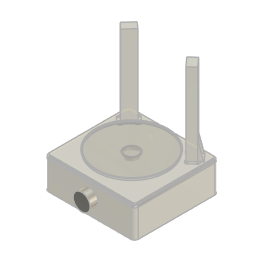
Elegoo Mercury X Cure Station (Autodesk Fusion 360 design; units mm, degrees)
Autodesk Fusion 360 part; units mm, degrees
sketch "Base" plane through (0, 0, 0) normal (0, 0, 1) x (1, 0, 0)
  line L0 (-113, 115) -> (113, 115)
  line L1 (123, 105) -> (123, -105)
  line L2 (113, -115) -> (-113, -115)
  line L3 (-123, -105) -> (-123, 105)
  arc A0 (-113, 115) -> (-123, 105) centre (-113, 105) ccw
  arc A1 (123, 105) -> (113, 115) centre (113, 105) ccw
  arc A2 (113, -115) -> (123, -105) centre (113, -105) ccw
  arc A3 (-123, -105) -> (-113, -115) centre (-113, -105) ccw
  line L4 (-113, 105) -> (113, -105) construction
  dimension "d1" = 10
  dimension "d7" = 246
  dimension "d8" = 230
  constraint horizontal L0
  constraint vertical L1
  constraint horizontal L2
  constraint vertical L3
  constraint tangent L0 A0
  constraint tangent L3 A0
  constraint tangent L0 A1
  constraint tangent L1 A1
  constraint equal A0 A1
  constraint tangent L1 A2
  constraint tangent L2 A2
  constraint equal A0 A2
  constraint tangent L2 A3
  constraint tangent L3 A3
  constraint equal A0 A3
  constraint coincident A0.centre L4.start
  constraint coincident A2.centre L4.end
  constraint midpoint origin L4
  measures "d1" radius of A0
  measures "d7" distance of L1 L3
  measures "d8" distance of L0 L2
extrude "Extrude1" add sketch "Base" along normal blind 81.5 makes body 1
sketch "Base Top" plane through (0, 0, 81.5) normal (0, 0, 1) x (-1, 0, 0)
  arc A0 (113, -115) -> (123, -105) centre (113, -105) ccw
  line L0 (123, -105) -> (123, 105)
  arc A1 (123, 105) -> (113, 115) centre (113, 105) ccw
  line L1 (113, 115) -> (-113, 115)
  arc A2 (-113, 115) -> (-123, 105) centre (-113, 105) ccw
  line L2 (-123, 105) -> (-123, -105)
  arc A3 (-123, -105) -> (-113, -115) centre (-113, -105) ccw
  line L3 (-113, -115) -> (113, -115)
  line L4 (113, 111) -> (-113, 111)
  arc A4 (-113, 111) -> (-119, 105) centre (-113, 105) ccw
  line L5 (-119, 105) -> (-119, -105)
  arc A5 (-119, -105) -> (-113, -111) centre (-113, -105) ccw
  line L6 (-113, -111) -> (113, -111)
  arc A6 (113, -111) -> (119, -105) centre (113, -105) ccw
  line L7 (119, -105) -> (119, 105)
  arc A7 (119, 105) -> (113, 111) centre (113, 105) ccw
  line L8 (113, 114.5) -> (-113, 114.5)
  arc A8 (-113, 114.5) -> (-122.5, 105) centre (-113, 105) ccw
  line L9 (-122.5, 105) -> (-122.5, -105)
  arc A9 (-122.5, -105) -> (-113, -114.5) centre (-113, -105) ccw
  line L10 (-113, -114.5) -> (113, -114.5)
  arc A10 (113, -114.5) -> (122.5, -105) centre (113, -105) ccw
  line L11 (122.5, -105) -> (122.5, 105)
  arc A11 (122.5, 105) -> (113, 114.5) centre (113, 105) ccw
  dimension "d53" = -0.5
  dimension "d54" = 3.5
  measures "d54" distance of L7 L11
extrude "Extrude2" add sketch "Base Top" along normal blind 4 contours L4 A4 L5 A5 L6 A6 L7 A7 bodies 1
extrude "Extrude8" cut sketch "Base Top" against normal blind 5.2 contours A0 L0 A1 L1 A2 L2 A3 L3 bodies 1
sketch "Wheel" plane through (0, -115, 0) normal (0, -1, 0) x (1, 0, 0)
  line L0 (-113, 0) -> (113, 0)
  line L1 (113, 0) -> (113, 76.3)
  line L2 (-113, 76.3) -> (-113, 0)
  circle A0 centre (0, 43.15) radius 23.35
  line L3 (0, 66.5) -> (0, 81.5) construction
  line L4 (113, 76.3) -> (-113, 76.3)
  dimension "d9" = 46.7
  dimension "d10" = 15
  constraint coincident A0 L3.start
  constraint vertical L3
  constraint coincident A0.centre L3
  measures "d9" diameter of A0
  measures "d10" distance of L3.start L3.end
extrude "Extrude3" add sketch "Wheel" along normal blind 22 contours A0 bodies 1
sketch "Plate" plane through (0, 0, 0) normal (0, 1, 0) x (1, 0, 0)
  line L0 (20.25, -81.275) -> (20.6, -94.275)
  line L1 (20.6, -94.275) -> (96.966, -94.275)
  line L2 (96.966, -94.275) -> (98.5, -100)
  line L3 (95.3809, -98.405) -> (0, -98.405)
  line L4 (0, -98.405) -> (0, -94.275)
  line L5 (0, -94.275) -> (17.4, -94.275)
  line L6 (17.4, -94.275) -> (17.75, -81.275)
  line L7 (17.75, -81.275) -> (20.25, -81.275)
  line L8 (98.5, -100) -> (95.8083, -100)
  line L9 (95.8083, -100) -> (95.3809, -98.405)
  line L10 (-113, -85.5) -> (113, -85.5)
  dimension "d14" = 98.5
  dimension "d16" = 2.6
  dimension "d17" = 5.725
  dimension "d18" = 4.13
  dimension "d20" = 20.6
  dimension "d23" = 20.25
  dimension "d24" = 2.5
  dimension "d25" = 13
  dimension "d27" = 75
  dimension "d28" = 14.5
  constraint perpendicular L3 L4
  constraint perpendicular L4 L5
  constraint horizontal L8
  constraint parallel L2 L9
  constraint horizontal L7
  constraint coincident L0.end L5
  constraint equal L0 L6
  constraint coincident origin L4
  measures "d14" distance of L4 L2.end
  measures "d16" distance of L2 L9
  measures "d17" distance of L1 L8
  measures "d18" distance of L1 L3
  measures "d20" distance of L0.end L4
  measures "d23" distance of L0.start L4
  measures "d24" distance of L0.start L6.end
  measures "d25" distance of L5.end L7
  measures "d27" angle of L1 L2
  measures "d28" distance of L8 L10
revolve "Revolve1" add sketch "Plate" angle 360 about axis through (0, 0, 98.405) along (0, 0, -1) separate body makes body 2
sketch "Tower" plane through (0, 0, 85.5) normal (0, 0, 1) x (-1, 0, 0)
  arc A0 (119, 105) -> (113, 111) centre (113, 105) ccw
  line L0 (113, 111) -> (-113, 111)
  arc A1 (-113, 111) -> (-119, 105) centre (-113, 105) ccw
  line L1 (-119, 105) -> (-119, -105)
  arc A2 (-119, -105) -> (-113, -111) centre (-113, -105) ccw
  line L2 (-113, -111) -> (113, -111)
  arc A3 (113, -111) -> (119, -105) centre (113, -105) ccw
  line L3 (119, -105) -> (119, 105)
  line L4 (89.4753, -59.2376) -> (106.3, -74.9248)
  line L5 (106.3, -74.9248) -> (84.3525, -99.3)
  line L6 (84.3525, -99.3) -> (66.9925, -84.2073)
  line L7 (66.9925, -84.2073) -> (89.4753, -59.2376)
  dimension "d30" = 32.8
  dimension "d31" = 33.6
  dimension "d32" = 23
  dimension "d33" = 12.7
  dimension "d34" = 11.7
  dimension "d36" = 42
  constraint parallel L5 L7
  constraint equal L4 L6
  measures "d30" distance of L4.end L5.end
  measures "d31" distance of L4.start L6.end
  measures "d32" distance of L5 L7
  measures "d33" distance of L3 L4.end
  measures "d34" distance of L2 L5.end
  measures "d36" angle of L3 L5
extrude "Extrude4" add sketch "Tower" along normal blind 225 separate body contours L4 L5 L6 L7 makes body 3
ref_plane "WorkPlane1" through (-86.6728, 79.3208, 198) normal (-0.669131, -0.743145, 0) x (0.743145, -0.669131, 0)
sketch "Tower Support" plane through (0.6366, 0.7071, 0) normal (-0.669131, -0.743145, 0) x (0.743145, -0.669131, 0)
  line L0 (-129.1308, 134.9) -> (-140.1308, 85.5)
  line L1 (-140.1308, 85.5) -> (-129.1308, 85.5)
  line L2 (-129.1308, 85.5) -> (-129.1308, 134.9)
  line L3 (-129.1308, 85.5) -> (-129.1308, 310.5)
  line L4 (-106.1308, 85.5) -> (-106.1308, 310.5)
  dimension "d39" = 34
  dimension "d40" = 49.4
  constraint horizontal L1
  constraint perpendicular L1 L2
  constraint coincident L0.start L3
  constraint coincident L1.end L2.start
  measures "d39" distance of L0.end L4
  measures "d40" distance of L0.start L1.end
extrude "Extrude5" add sketch "Tower Support" along normal mid plane 29 bodies 3
extrude "Extrude6" cut sketch "Tower Support" along normal mid plane 25.5 bodies 1 3
sketch "Tower Base" plane through (0, 0, 85.5) normal (0, 0, -1) x (1, 0, 0)
  line L0 (-112.0323, -84.9978) -> (-103.8577, -77.6373)
  line L1 (-103.8577, -77.6373) -> (-86.7948, -96.5875)
  line L2 (-86.7948, -96.5875) -> (-94.9694, -103.948)
  line L3 (-94.9694, -103.948) -> (-93.7985, -105.2485)
  line L4 (-93.7985, -105.2485) -> (-85.6239, -97.888)
  line L5 (-85.6239, -97.888) -> (-84.3525, -99.3)
  line L6 (-84.3525, -99.3) -> (-66.9925, -84.2073)
  line L7 (-66.9925, -84.2073) -> (-89.4753, -59.2376)
  line L8 (-89.4753, -59.2376) -> (-106.3, -74.9248)
  line L9 (-106.3, -74.9248) -> (-105.0287, -76.3368)
  line L10 (-105.0287, -76.3368) -> (-113.2032, -83.6973)
  line L11 (-113.2032, -83.6973) -> (-112.0323, -84.9978)
  line L12 (-93.84, -85.7742) -> (-88.3196, -91.9051)
  line L13 (-84.0828, -92.1272) -> (-71.0778, -80.4174)
  line L14 (-66.841, -80.6394) -> (-62.3578, -85.6185)
  line L15 (-62.5798, -89.8553) -> (-80.4153, -105.9144)
  line L16 (-84.6521, -105.6924) -> (-85.6224, -104.6148)
  line L17 (-89.8592, -104.3928) -> (-91.3455, -105.7311)
  line L18 (-95.5823, -105.509) -> (-104.6156, -95.4766)
  line L19 (-104.6156, -95.4766) -> (-93.84, -85.7742)
  circle A0 centre (-66.3041, -87.9607) radius 1.7
  circle A1 centre (-81.9102, -102.0125) radius 1.7
  circle A2 centre (-101.2714, -92.4655) radius 1.7
  line L20 (-81.9102, -102.0125) -> (-66.3041, -87.9607) construction
  arc A3 (-95.5823, -105.509) -> (-91.3455, -105.7311) centre (-93.3529, -103.5016) ccw
  arc A4 (-85.6224, -104.6148) -> (-89.8592, -104.3928) centre (-87.8518, -106.6222) ccw
  arc A5 (-84.6521, -105.6924) -> (-80.4153, -105.9144) centre (-82.4227, -103.685) ccw
  arc A6 (-62.5798, -89.8553) -> (-62.3578, -85.6185) centre (-64.5872, -87.6259) ccw
  arc A7 (-66.841, -80.6394) -> (-71.0778, -80.4174) centre (-69.0704, -82.6468) ccw
  arc A8 (-88.3196, -91.9051) -> (-84.0828, -92.1272) centre (-86.0902, -89.8977) ccw
  point P0 (-86.3122, -94.1345)
  point P1 (-60.3504, -87.8479)
  point P2 (-82.6447, -107.9218)
  point P3 (-93.5749, -107.7384)
  point P4 (-95.3263, -87.1124)
  dimension "d57" = 12.7
  dimension "d58" = 14.5
  dimension "d59" = 12.5
  dimension "d60" = 38
  dimension "d61" = 11.25
  dimension "d62" = 16.5
  dimension "d63" = 30
  dimension "d64" = 3.4
  dimension "d65" = 4.5
  dimension "d66" = 3.9
  dimension "d67" = 21
  dimension "d68" = 4.5
  dimension "d69" = 3
  constraint perpendicular L2 L12
  constraint perpendicular L7 L13
  constraint perpendicular L2 L14
  constraint perpendicular L7 L15
  constraint perpendicular L2 L16
  constraint perpendicular L16 L17
  constraint perpendicular L2 L18
  constraint midpoint L1 P4
  constraint coincident L19 P4
  constraint perpendicular L1 L19
  constraint coincident L19 A2.centre
  constraint equal A1 A2
  constraint equal A0 A1
  constraint coincident A1.centre L20.start
  constraint coincident A0.centre L20.end
  constraint parallel L15 L20
  constraint coincident P3 L17
  constraint coincident P3 L18
  constraint tangent L17 A3
  constraint tangent L18 A3
  constraint tangent L16 A4
  constraint tangent L17 A4
  constraint equal A3 A4
  constraint coincident P2 L15
  constraint coincident P2 L16
  constraint tangent L15 A5
  constraint tangent L16 A5
  constraint equal A3 A5
  constraint coincident P1 L14
  constraint coincident P1 L15
  constraint tangent L14 A6
  constraint tangent L15 A6
  constraint equal A3 A6
  constraint tangent L13 A7
  constraint tangent L14 A7
  constraint equal A3 A7
  constraint coincident P0 L12
  constraint coincident P0 L13
  constraint tangent L12 A8
  constraint tangent L13 A8
  constraint equal A3 A8
  measures "d57" distance of L13 L15
  measures "d58" distance of L12.start L18.end
  measures "d59" distance of L1 L18
  measures "d60" distance of L14 L18
  measures "d61" distance of L12.start P0
  measures "d62" distance of P3 L18.end
  measures "d63" distance of P1 P2
  measures "d64" diameter of A0
  measures "d65" distance of L14 A0.centre
  measures "d66" distance of L15 A0.centre
  measures "d67" distance of A0.centre A1.centre
  measures "d68" distance of L18 A2.centre
  measures "d69" radius of A3
extrude "Extrude9" add sketch "Tower Base" along normal blind 2 contours L1 L2 L3 L4 L5 L6 L7 L12 L13 L19 A7 A8 | L1 L2 L3 L4 L5 L6 L7 L14 L15 L16 L17 L18 L19 A2 A3 A4 A5 A6 A7 bodies 3
mirror "Mirror2" about plane through (-95.3263, 87.1124, 85.5) normal (-0.669131, -0.743145, 0) of "Extrude9"
mirror "Mirror1" about plane through (0, 0, 0) normal (1, 0, 0) of bodies 3 makes body 4
sketch "Power Port" plane through (0, 115, 0) normal (0, 1, 0) x (-1, 0, 0)
  line L0 (-113, 0) -> (113, 0)
  line L1 (113, 0) -> (113, 76.3)
  line L2 (-113, 76.3) -> (-113, 0)
  circle A0 centre (62.75, 39.95) radius 6.25
  line L3 (62.75, 46.2) -> (62.75, 81.5) construction
  line L4 (69, 39.95) -> (123, 39.95) construction
  line L5 (123, 0) -> (123, 76.3) construction
  circle A1 centre (62.75, 39.95) radius 2.8
  line L6 (113, 76.3) -> (-113, 76.3)
  line L7 (113, 81.5) -> (-113, 81.5)
  dimension "d47" = 12.5
  dimension "d48" = 35.3
  dimension "d49" = 54
  dimension "d50" = 5.6
  constraint coincident A0 L3.start
  constraint coincident A0.centre L3
  constraint coincident A0 L4.start
  constraint horizontal L4
  constraint coincident L4.end L5
  constraint coincident A0.centre L4
  constraint concentric A0 A1
  constraint coincident L3.end L7
  measures "d47" diameter of A0
  measures "d48" distance of L3.start L3.end
  measures "d49" distance of L4.start L4.end
  measures "d50" diameter of A1
extrude "Extrude7" add sketch "Power Port" along normal blind 2.1 contours A0 bodies 1 3
equation "d14 = ( 197 / 2 ) * 1 mm"
equation "d20 = ( 41.2 / 2 ) * 1 mm"
equation "d23 = ( 40.5 / 2 ) * 1 mm"
equation "d61 = ( 22.5 / 2 ) * 1 mm"
equation "d62 = ( 33 / 2 ) * 1 mm"
equation "d66 = 2.2 mm + ( 3.4 / 2 ) * 1 mm"
equation "d67 = 17.6 mm + 3.4 mm"
named bodies: "Main", "Plate", "Tower L", "Tower R"
